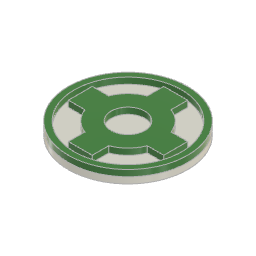
_Roundabout.ea690ca7-36d7-46e8-882e-ac7acc4cefcd (Autodesk Fusion 360 design; units mm, degrees)
Autodesk Fusion 360 part; units mm, degrees
sketch "Sketch1" plane through (0, 0, 0) normal (0, 0, 1) x (1, 0, 0)
  circle A0 centre (0, 0) radius 15.875
  circle A1 centre (0, 0) radius 14.2875
  line L0 (0, 12.7) -> (3.175, 12.7)
  line L1 (3.175, 0) -> (0, 0)
  line L2 (0, 0) -> (3.175, 0)
  line L3 (3.175, -12.7) -> (0, -12.7)
  line L4 (0, -12.7) -> (-3.175, -12.7)
  line L5 (-3.175, 12.7) -> (0, 12.7)
  line L6 (12.7, 0) -> (12.7, 3.175)
  line L7 (0, 3.175) -> (0, 0)
  line L8 (12.7, 0) -> (12.7, -3.175)
  line L9 (0, -3.175) -> (0, 0)
  line L10 (-12.7, 3.175) -> (-12.7, -3.175)
  circle A2 centre (0, 0) radius 8.89
  circle A3 centre (0, 0) radius 4.4901
  line L11 (3.175, -8.3037) -> (3.175, -12.7)
  line L12 (3.175, -12.7) -> (-3.175, -12.7)
  line L13 (-3.175, -12.7) -> (-3.175, -8.3037)
  line L14 (-12.7, 3.175) -> (-8.3037, 3.175)
  line L15 (-8.3037, -3.175) -> (-12.7, -3.175)
  line L16 (-12.7, -3.175) -> (-12.7, 3.175)
  line L17 (-3.175, 12.7) -> (3.175, 12.7)
  line L18 (3.175, 12.7) -> (3.175, 8.3037)
  line L19 (3.175, 8.3037) -> (-3.175, 8.3037)
  line L20 (-3.175, 8.3037) -> (-3.175, 12.7)
  line L21 (12.7, 3.175) -> (8.3037, 3.175)
  line L22 (8.3037, -3.175) -> (12.7, -3.175)
  line L23 (12.7, -3.175) -> (12.7, 3.175)
  dimension "d1" = 31.75
  dimension "d2" = 28.575
  dimension "d3" = 3.175
  dimension "d4" = 12.7
  dimension "d5" = 3.175
  dimension "d6" = 12.7
  dimension "d7" = 3.175
  dimension "d8" = 3.175
  dimension "d9" = 12.7
  constraint coincident A0.centre A1.centre
  constraint concentric A0 A1
  constraint horizontal L0
  constraint horizontal L1
  constraint horizontal L2
  constraint horizontal L3
  constraint horizontal L4
  constraint horizontal L5
  constraint vertical L6
  constraint vertical L7
  constraint vertical L8
  constraint vertical L9
  constraint vertical L10
  constraint concentric A1 A2
  constraint concentric A1 A3
  constraint vertical L11
  constraint horizontal L12
  constraint vertical L13
  constraint coincident A2 L13.end
  constraint horizontal L14
  constraint horizontal L15
  constraint vertical L16
  constraint coincident A2 L15.start
  constraint horizontal L17
  constraint vertical L18
  constraint horizontal L19
  constraint vertical L20
  constraint coincident A2 L18.end
  constraint horizontal L21
  constraint horizontal L22
  constraint vertical L23
  constraint coincident A2 L22.start
  measures "d1" diameter of A0
  measures "d2" diameter of A1
  measures "d3" distance of L0.start L0.end
  measures "d4" distance of A0.centre L3.end
  measures "d5" distance of L3.end L4.end
  measures "d6" distance of A0.centre L6.start
  measures "d7" distance of A0.centre L7.start
  measures "d8" distance of A0.centre L9.start
  measures "d9" distance of L7.start L10.start
extrude "Extrude1" add sketch "Sketch1" along normal blind 1 makes body 1 at (15.2335, -1.4985, 0) makes body 2 at (-1.0583, 11.2346, 0) in component "Component"
extrude "Extrude3" add sketch "Sketch1" against normal blind 1 separate body contours A0 | A1 | L0 L5 A2 L17 L18 L20 | A2 L19 | A2 L19 | L6 L8 A2 L21 L22 L23 | L10 A2 L14 L15 L16 | L3 L4 A2 L11 L12 L13 | A3 makes body 3
scale "Scale1" factors (0.6, 0.6, 1) about (-4.4901, 0, 1) bodies 2 1 in component "Component"
scale "Scale1'" factors (0.6, 0.6, 1) about (-4.4901, 0, 1) bodies 3
component "Component" placed x (1, 0, 0) y (0, 1, 0) z (0, 0, 1) at (0, 0, 0)
